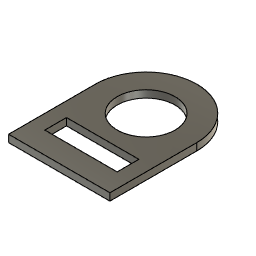
e1 (Autodesk Fusion 360 design; units mm, degrees)
Autodesk Fusion 360 part; units mm, degrees
sketch "Sketch1" plane through (0, 0, 0) normal (0, 0, 1) x (1, 0, 0)
  line L0 (0, 0) -> (70, 0)
  line L1 (70, 0) -> (70, 60)
  line L2 (0, 60) -> (0, 0)
  line L3 (10, 15) -> (60, 15)
  line L4 (60, 15) -> (60, 30)
  line L5 (60, 30) -> (10, 30)
  line L6 (10, 30) -> (10, 15)
  circle A0 centre (35, 60) radius 20
  arc A1 (70, 60) -> (0, 60) centre (35, 60) ccw
  dimension "d1" = 70
  dimension "d2" = 60
  dimension "d5" = 15
  dimension "d6" = 50
  dimension "d10" = 10
  dimension "d11" = 15
  dimension "d15" = 40
  dimension "d16" = 35
  constraint horizontal L0
  constraint vertical L1
  constraint vertical L2
  constraint coincident L0.start L2.end
  constraint horizontal L3
  constraint vertical L4
  constraint horizontal L5
  constraint vertical L6
  constraint tangent L1 A1
  measures "d1" distance of L0.start L0.end
  measures "d2" distance of L0.start L2.start
  measures "d5" distance of L3.end L4.end
  measures "d6" distance of L4.end L5.end
  measures "d10" distance of L2 L6
  measures "d11" distance of L0 L3
  measures "d15" diameter of A0
  measures "d16" radius of A1
extrude "Extrude1" add sketch "Sketch1" along normal blind 5
